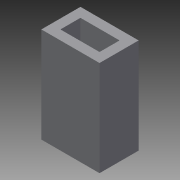
# Autodesk Inventor part: HammerStick Sleeve
Saved by Autodesk Inventor 2015 (Build 190159000, 159)
## iProperties
Created: 2015-01-13
Part Number: HammerStick Sleeve
Material: Generic
Document SubType Name: Modeling
Designer: harrykuperstein
Density: 1 g/cm^3
Appearance: Default
Author: harrykuperstein
Autodesk Inventor part; units mm, degrees
ref_plane "YZ Plane" through (0, 0, 0) normal (1, 0, 0) x (0, 1, 0)
ref_plane "XZ Plane" through (0, 0, 0) normal (0, 1, 0) x (-1, 0, 0)
ref_plane "XY Plane" through (0, 0, 0) normal (0, 0, 1) x (1, 0, 0)
sketch "Sketch1" plane through (0, 0, 0) normal (0, 1, 0) x (-1, 0, 0)
  line L0 (0, 0) -> (52.07, 0)
  line L1 (52.07, 0) -> (52.07, 26.67)
  line L2 (52.07, 26.67) -> (0, 26.67)
  line L3 (0, 26.67) -> (0, 0)
  line L4 (-12.7, 39.37) -> (64.77, 39.37)
  line L5 (64.77, 39.37) -> (64.77, -12.7)
  line L6 (64.77, -12.7) -> (-12.7, -12.7)
  line L7 (-12.7, -12.7) -> (-12.7, 39.37)
  dimension "d0" = 26.67
  dimension "d1" = 52.07
  dimension "d2" = 12.7
  dimension "d3" = 12.7
  dimension "d4" = 12.7
  dimension "d5" = 12.7
  constraints: 16 end point, 4 parallel, 2 horizontal, 2 perpendicular
  measures "d0" distance of L2.end L0.start
  measures "d1" distance of L0.start L0.end
  measures "d2" distance between parallel lines of L2 L4
  measures "d3" distance between parallel lines of L6 L0
  measures "d4" distance between parallel lines of L1 L5
  measures "d5" distance between parallel lines of L7 L3
extrude "Extrusion1" add sketch "Sketch1" along normal blind 127
sketch "Sketch2" plane through (0, 0, 0) normal (0, -1, 0) x (1, 0, 0)
  line L0 (0, 0) -> (-52.07, 0)
  line L1 (-52.07, 0) -> (-52.07, 26.67)
  line L2 (-52.07, 26.67) -> (0, 26.67)
  line L3 (0, 26.67) -> (0, 0)
  constraints: 8 end point, 2 parallel, 1 horizontal, 1 perpendicular
extrude "Extrusion2" add sketch "Sketch2" against normal blind 5.08
body "Solid1"
